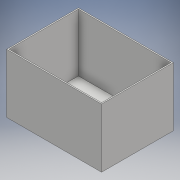
# Autodesk Inventor part: Startup for arduino board
Saved by Autodesk Inventor 2018 (Build 220112000, 112)
## iProperties
Created: 2018-04-25
Part Number: Startup for arduino board
Material: Generic
Document SubType Name: Modeling
Designer: Sebastian Carlsson
Density: 1 g/cm^3
Appearance: Default
Author: Sebastian Carlsson
Autodesk Inventor part; units mm, degrees
ref_plane "YZ Plane" through (0, 0, 0) normal (1, 0, 0) x (0, 1, 0)
ref_plane "XZ Plane" through (0, 0, 0) normal (0, 1, 0) x (-1, 0, 0)
ref_plane "XY Plane" through (0, 0, 0) normal (0, 0, 1) x (1, 0, 0)
sketch "Sketch1" plane through (0, 0, 0) normal (0, 0, 1) x (1, 0, 0)
  line L0 (0, 0) -> (80, 0) construction
  line L1 (0, 0) -> (80, 0)
  line L2 (80, 0) -> (80, -60)
  line L3 (80, -60) -> (0, -60)
  line L4 (0, -60) -> (0, 0)
  dimension "d2" = 80
  dimension "d3" = 60
  constraints: 10 end point, 2 horizontal, 2 parallel, 1 perpendicular
  measures "d2" distance of L2.end L3.end
  measures "d3" distance of L1.end L2.end
extrude "Extrusion1" add sketch "Sketch1" along normal blind 50
shell "Shell1" thickness 1 outward yes removed faces 1 at (26.6667, -20, 50)
sketch "Sketch2" plane through (0, 0, 0) normal (0, 0, 1) x (1, 0, 0)
  circle A0 centre (2, -40) radius 1
  point P0 (0, 0)
  dimension "d7" = 2
  constraints: 1 centre point
  measures "d7" diameter of A0
hole "Hole1" at (2, -40, 0) direction (0, 0, -1) diameter 2 end through all
sketch "Sketch3" plane through (0, 0, 0) normal (0, 0, 1) x (1, 0, 0)
  circle A0 centre (2, -13) radius 1
  point P0 (0, 0)
  dimension "d15" = 2
  constraints: 1 centre point
  measures "d15" diameter of A0
hole "Hole2" at (2, -13, 0) direction (0, 0, -1) diameter 2 end through all
body "Solid1"
